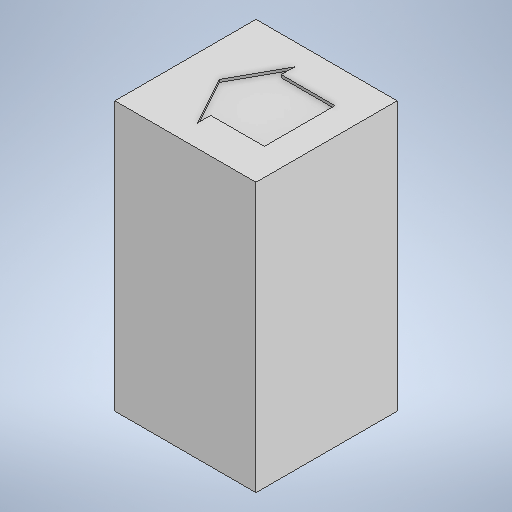
# Autodesk Inventor part: Air_heater_button
Saved by Autodesk Inventor 2025.2 (Build 292293000, 293)
## iProperties
Created: 2025-09-19
Part Number: Air_heater_button
Material: Generic
Document SubType Name: Modeling
Designer: TSO
Density: 1 g/cm^3
Appearance: Default
Author: TSO
Autodesk Inventor part; units mm, degrees
ref_plane "YZ Plane" through (0, 0, 0) normal (1, 0, 0) x (0, 1, 0)
ref_plane "XZ Plane" through (0, 0, 0) normal (0, 1, 0) x (-1, 0, 0)
ref_plane "XY Plane" through (0, 0, 0) normal (0, 0, 1) x (1, 0, 0)
sketch "Sketch1" plane through (0, 0, 0) normal (0, 1, 0) x (-1, 0, 0)
  line L0 (0, 0) -> (10.5, 0)
  line L1 (10.5, 0) -> (10.5, -10.5)
  line L2 (10.5, -10.5) -> (0, -10.5)
  line L3 (0, -10.5) -> (0, 0)
  dimension "d0" = 10.5
  dimension "d1" = 10.5
  constraints: 8 end point, 2 parallel, 1 horizontal, 1 perpendicular
  measures "d0" distance of L1.end L2.end
  measures "d1" distance of L0.end L1.end
extrude "Extrusion1" add sketch "Sketch1" along normal blind 20
sketch "Sketch2" plane through (0, 20, 0) normal (0, 1, 0) x (1, 0, 0)
  line L0 (0, 0) -> (-2, 0)
  line L1 (-2, 0) -> (-2, 2.625)
  line L2 (-2, 2.625) -> (0, 2.625)
  line L3 (0, 2.625) -> (0, 0)
  line L4 (-2, 2.625) -> (-6, 2.625)
  line L5 (-6, 2.625) -> (-6, 7.875)
  line L6 (-6, 7.875) -> (-2, 7.875)
  line L7 (-2, 7.875) -> (-2, 2.625)
  line L8 (-6, 2.625) -> (-8, 2.625) construction
  line L9 (-8, 2.625) -> (-8, 1.625) construction
  line L10 (-8, 1.625) -> (-6, 1.625) construction
  line L11 (-6, 1.625) -> (-6, 2.625)
  line L12 (-6, 1.625) -> (-8, 1.625)
  line L13 (-8, 1.625) -> (-8, 8.875) construction
  line L14 (-8, 8.875) -> (-6, 8.875)
  line L15 (-6, 8.875) -> (-6, 1.625)
  line L16 (-8, 5.25) -> (-6, 1.625)
  line L17 (-8, 5.25) -> (-6, 8.875)
  dimension "d4" = 2
  dimension "d5" = 2.625
  dimension "d6" = 4
  dimension "d7" = 5.25
  dimension "d8" = 2
  dimension "d9" = 1
  dimension "d10" = 2
  dimension "d11" = 7.25
  constraints: 36 end point, 8 parallel, 4 horizontal, 4 perpendicular, 1 midpoint
  measures "d4" distance of L1.end L2.end
  measures "d5" distance of L0.end L1.end
  measures "d6" distance of L5.end L6.end
  measures "d7" distance of L4.end L5.end
  measures "d8" distance of L10.end L9.end
  measures "d9" distance of L9.end L8.end
  measures "d10" distance of L13.end L14.end
  measures "d11" distance of L12.end L13.end
extrude "Extrusion2" cut sketch "Sketch2" against normal blind 0.2 contours L4 L5 L6 L7 | L11 L16 L17 L15 L5
body "Solid1"
